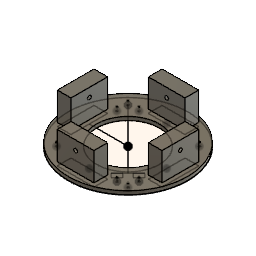
top_joint_print v3 (Autodesk Fusion 360 design; units mm, degrees)
Autodesk Fusion 360 part; units mm, degrees
sketch "Sketch1" plane through (0, 0, 0) normal (0, 1, 0) x (1, 0, 0)
  circle A0 centre (0, 0) radius 17.095
  circle A1 centre (0, 0) radius 32.5
  line L0 (-21.05, 10) -> (-28.55, 10)
  line L1 (-28.55, 10) -> (-28.55, -10)
  line L2 (-28.55, -10) -> (-21.05, -10)
  line L3 (-21.05, -10) -> (-21.05, 10)
  line L4 (-21.05, 0) -> (0, 0)
  line L5 (0, 0) -> (-19.4454, 19.4454)
  circle A2 centre (-19.4454, 19.4454) radius 0.5
  line L6 (-10, -21.05) -> (-10, -28.55)
  line L7 (10, -28.55) -> (10, -21.05)
  line L8 (-10, -28.55) -> (10, -28.55)
  line L9 (10, -21.05) -> (-10, -21.05)
  circle A3 centre (-19.4454, -19.4454) radius 0.5
  line L10 (21.05, -10) -> (28.55, -10)
  line L11 (28.55, 10) -> (21.05, 10)
  line L12 (28.55, -10) -> (28.55, 10)
  line L13 (21.05, 10) -> (21.05, -10)
  circle A4 centre (19.4454, -19.4454) radius 0.5
  line L14 (10, 21.05) -> (10, 28.55)
  line L15 (-10, 28.55) -> (-10, 21.05)
  line L16 (10, 28.55) -> (-10, 28.55)
  line L17 (-10, 21.05) -> (10, 21.05)
  circle A5 centre (19.4454, 19.4454) radius 0.5
  line L18 (17.3241, -8.1317) -> (8.1317, -17.3241)
  line L19 (0, 0) -> (12.7279, -12.7279)
  line L20 (10.253, -19.4454) -> (8.1317, -17.3241)
  line L21 (8.1317, -17.3241) -> (11.3137, -14.1421)
  line L22 (11.3137, -14.1421) -> (13.435, -16.2635)
  line L23 (13.435, -16.2635) -> (10.253, -19.4454)
  line L24 (19.4454, -10.253) -> (17.3241, -8.1317)
  line L25 (17.3241, -8.1317) -> (14.1421, -11.3137)
  line L26 (14.1421, -11.3137) -> (16.2635, -13.435)
  line L27 (16.2635, -13.435) -> (19.4454, -10.253)
  line L28 (11.844, -17.8544) -> (13.6118, -19.6222)
  circle A6 centre (13.6118, -19.6222) radius 0.5
  line L29 (17.8544, -11.844) -> (19.6222, -13.6118)
  circle A7 centre (19.6222, -13.6118) radius 0.5
  circle A8 centre (-13.6118, 19.6222) radius 0.5
  circle A9 centre (-19.6222, 13.6118) radius 0.5
  point P0 (0, -21.05)
  point P1 (21.05, 0)
  point P2 (0, 21.05)
  dimension "d1" = 34.19
  dimension "d2" = 65
  dimension "d4" = 21.05
  dimension "d5" = 20
  dimension "d6" = 7.5
  dimension "d7" = 27.5
  dimension "d8" = 1
  dimension "d9" = 45
  dimension "d11" = 360
  dimension "d13" = 13
  dimension "d14" = 18
  dimension "d15" = 3
  dimension "d16" = 4.5
  dimension "d17" = 3
  dimension "d18" = 4.5
  dimension "d19" = 2.5
  dimension "d20" = 1
  dimension "d21" = 2.5
  dimension "d22" = 1
  dimension "d24" = 360
  measures "d1" diameter of A0
  measures "d2" diameter of A1
  measures "d4" distance of L4.start A0.centre
  measures "d5" distance of L0.start L2.end
  measures "d6" distance of L0.start L0.end
  measures "d7" distance of A0.centre L5.end
  measures "d8" diameter of A2
  measures "d9" angle of L4 L5
  measures "d13" distance of L18.start L18.end
  measures "d14" distance of A0.centre L19.end
  measures "d15" distance of L18.end L20.start
  measures "d16" distance of L20.start L22.end
  measures "d17" distance of L18.start L24.start
  measures "d18" distance of L24.start L26.end
  measures "d19" distance of L28.start L28.end
  measures "d20" diameter of A6
  measures "d21" distance of L29.start L29.end
  measures "d22" diameter of A7
extrude "Extrude1" add sketch "Sketch1" along normal blind 12.45 contours L0 L1 L2 L3 | L6 L7 L8 L9 | L10 L11 L12 L13 | L14 L15 L16 L17 makes body 1 at (3.3333, 4.15, 21.05) makes body 2 at (21.05, 4.15, -3.3333) makes body 3 at (-21.05, 4.15, 3.3333) makes body 4 at (-3.3333, 4.15, -21.05)
extrude "Extrude2" add sketch "Sketch1" along normal blind 2 contours A1 | L18 L24 L25 L26 L27 | L18 L20 L21 L22 L23 bodies 1 2 3 4
extrude "Extrude3" add 4 faces at (-26.05, 12.45, 3.3333) (-3.3333, 12.45, 23.55) (23.55, 12.45, -3.3333) (3.3333, 12.45, -23.55) along direction (0, 1, 0) blind 1.8 on bodies 1 bodies 1
sketch "Sketch2" plane through (0, 0, 28.55) normal (0, 0, 1) x (1, 0, 0)
  line L0 (-10, 2) -> (10, 2)
  line L1 (10, 2) -> (10, 14.25)
  line L2 (10, 14.25) -> (-10, 14.25)
  line L3 (-10, 14.25) -> (-10, 2)
  circle A0 centre (0, 12.245) radius 1
  dimension "d31" = 2
  dimension "d32" = 12.245
  measures "d31" diameter of A0
  measures "d32" distance of origin A0.centre
extrude "Extrude4" add 4 faces at (-3.3333, 14.25, 23.55) (23.55, 14.25, -3.3333) (3.3333, 14.25, -23.55) (-26.05, 14.25, 3.3333) along direction (0, 1, 0) blind 3 on bodies 1 bodies 1
sketch "Sketch3" plane through (28.55, 0, 0) normal (1, 0, 0) x (0, 0, -1)
  line L0 (-10, 2) -> (10, 2)
  line L1 (10, 2) -> (10, 17.25)
  line L2 (10, 17.25) -> (-10, 17.25)
  line L3 (-10, 17.25) -> (-10, 2)
  circle A0 centre (0, 12.445) radius 1
  dimension "d35" = 2
  dimension "d36" = 12.445
  measures "d35" diameter of A0
  measures "d36" distance of origin A0.centre
extrude "Extrude5" cut sketch "Sketch3" against normal blind 60 contours A0 bodies 1
extrude "Extrude6" cut sketch "Sketch2" against normal blind 60 contours A0 bodies 1
